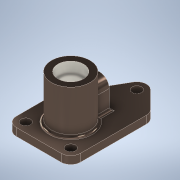
# Autodesk Inventor part: Part12. Pole Foot
Saved by Autodesk Inventor 2022.2 (Build 262287010, 287A)
## iProperties
Created: 2022-12-07
Part Number: Part12. Pole Foot
Material: Steel, Carbon
Document SubType Name: Modeling
Designer: User
Mass: 2300.87 g
Surface Area: 538.828 cm^2
Volume: 293.105 cm^3
Density: 7.85 g/cm^3
Appearance: Gunmetal - Antique Polished
Author: User
Autodesk Inventor part; units mm, degrees
ref_plane "YZ Plane" through (0, 0, 0) normal (1, 0, 0) x (0, 1, 0)
ref_plane "XZ Plane" through (0, 0, 0) normal (0, 1, 0) x (-1, 0, 0)
sketch "Sketch2" plane through (0, 0, 0) normal (0, 1, 0) x (-1, 0, 0)
  circle A0 centre (0, 0) radius 15
  line L0 (35, 50) -> (-35, 50)
  line L1 (-50, 35) -> (-50, -68)
  line L2 (50, -20.5218) -> (50, 35)
  circle A1 centre (-8, -95) radius 7.5
  arc A2 (-18.6066, -105.6066) -> (4.9904, -102.5) centre (-8, -95) ccw
  line L3 (-18.6066, -105.6066) -> (-45.6066, -78.6066)
  line L4 (-18.6066, -105.6066) -> (19.5772, -105.6066) construction
  line L5 (4.9904, -102.5) -> (47.9904, -28.0218)
  line L6 (4.9904, -102.5) -> (90.9904, -102.5) construction
  arc A3 (-50, -68) -> (-45.6066, -78.6066) centre (-35, -68) ccw
  arc A4 (47.9904, -28.0218) -> (50, -20.5218) centre (35, -20.5218) ccw
  arc A5 (-35, 50) -> (-50, 35) centre (-35, 35) ccw
  arc A6 (50, 35) -> (35, 50) centre (35, 35) ccw
  circle A7 centre (35, 35) radius 7.5
  circle A8 centre (-35, 35) radius 7.5
  dimension "d11" = 30
  dimension "d12" = 50
  dimension "d13" = 50
  dimension "d14" = 100
  dimension "d15" = 15
  dimension "d16" = 145
  dimension "d17" = 42
  dimension "d19" = 60
  dimension "d21" = 15
  dimension "d22" = 135
  dimension "d23" = 15
  dimension "d24" = 15
  dimension "d25" = 15
  constraints: 14 end point, 12 point on circle, 10 tangent, 9 centre point, 4 coincident, 3 equal radius, 3 horizontal, 2 equal length, 2 point on line, 1 parallel, 1 perpendicular
  measures "d11" diameter of A0
  measures "d12" distance from line of point (0, 0) L0
  measures "d13" distance from line of L2 point (0, 0)
  measures "d14" distance between parallel lines of L1 L2
  measures "d15" diameter of A1
  measures "d16" distance from line of A1.centre L0
  measures "d17" distance from line of L1 A1.centre
  measures "d19" angle of L6 L5
  measures "d21" radius of A2
  measures "d22" angle of L1 L3
  measures "d23" radius of A3
  measures "d24" diameter of A7
  measures "d25" diameter of A8
extrude "Extrusion1" add sketch "Sketch2" along normal blind 12
sketch "Sketch3" plane through (0, 12, 0) normal (0, 1, 0) x (1, 0, 0)
  circle A0 centre (0, 0) radius 15 projected
  line L0 (-4.9904, 102.5) -> (-47.9904, 28.0218) projected
  arc A1 (-47.9904, 28.0218) -> (-50, 20.5218) centre (-35, 20.5218) ccw projected
  line L1 (-50, 20.5218) -> (-50, -35) projected
  arc A2 (-50, -35) -> (-35, -50) centre (-35, -35) ccw projected
  line L2 (-35, -50) -> (35, -50) projected
  arc A3 (35, -50) -> (50, -35) centre (35, -35) ccw projected
  line L3 (50, -35) -> (50, 68) projected
  arc A4 (50, 68) -> (45.6066, 78.6066) centre (35, 68) ccw projected
  line L4 (45.6066, 78.6066) -> (18.6066, 105.6066) projected
  arc A5 (18.6066, 105.6066) -> (-4.9904, 102.5) centre (8, 95) ccw projected
  circle A6 centre (0, 0) radius 15 projected
  circle A7 centre (35, -35) radius 7.5 projected
  circle A8 centre (-35, -35) radius 7.5 projected
  circle A9 centre (8, 95) radius 7.5 projected
  circle A10 centre (0, 0) radius 30
  dimension "d28" = 60
  constraints: 1 centre point, 1 coincident
  measures "d28" diameter of A10
extrude "Extrusion2" add sketch "Sketch3" along normal blind 68 contours A10
sketch "Sketch4" plane through (0, 80, 0) normal (0, 1, 0) x (1, 0, 0)
  circle A0 centre (0, 0) radius 15 projected
  circle A1 centre (0, 0) radius 30 projected
  circle A2 centre (0, 0) radius 15 projected
  circle A3 centre (0, 0) radius 20
  dimension "d31" = 40
  constraints: 1 centre point, 1 coincident
  measures "d31" diameter of A3
extrude "Extrusion3" cut sketch "Sketch4" against normal blind 16 contours A3
ref_plane "Work Plane1" through (0, 0, -30) normal (0, 0, 1) x (1, 0, 0)
sketch "Sketch5" plane through (0, 0, -30) normal (0, 0, 1) x (1, 0, 0)
  line L0 (0, -16) -> (0, 96) construction
  line L1 (-70, 0) -> (70, 0) construction
  circle A0 centre (0, 42) radius 8
  arc A1 (15, 42) -> (-15, 42) centre (0, 42) ccw
  line L2 (-35, 0) -> (35, 0) projected
  line L3 (35, 0) -> (35, 12) projected
  line L4 (-35, 12) -> (35, 12) projected
  line L5 (-35, 0) -> (-35, 12) projected
  line L6 (15, 42) -> (15, 12)
  line L7 (-15, 42) -> (-15, 12)
  point P0 (0, 0)
  point P1 (0, 57)
  dimension "d35" = 16
  dimension "d36" = 42
  dimension "d37" = 15
  constraints: 4 end point, 4 point on line, 3 point on circle, 2 centre point, 2 perpendicular, 2 tangent, 1 coincident
  measures "d35" diameter of A0
  measures "d36" distance from line of L1 A0.centre
  measures "d37" radius of A1
extrude "Extrusion4" add sketch "Sketch5" along normal up to surface contours L6 L4 L7 A1 round surface about axis through (0, 12, 0) along (0, 1, 0) radius 30 far side no
sketch "Sketch6" plane through (0, 0, -30) normal (0, 0, -1) x (-1, 0, 0)
  arc A0 (0, 57) -> (-15, 42) centre (0, 42) ccw projected
  line L0 (-15, 12) -> (-15, 42) projected
  line L1 (15, 12) -> (-15, 12) projected
  line L2 (15, 42) -> (15, 12) projected
  arc A1 (15, 42) -> (0, 57) centre (0, 42) ccw projected
  arc A2 (0, 34) -> (0, 50) centre (0, 42) ccw projected
  arc A3 (0, 34) -> (0, 50) centre (0, 42) ccw projected
  point P0 (0, 0)
extrude "Extrusion5" add sketch "Sketch6" along normal blind 15
sketch "Sketch7" plane through (0, 0, -45) normal (0, 0, -1) x (-1, 0, 0)
  arc A0 (15, 42) -> (-15, 42) centre (0, 42) ccw projected
  arc A1 (15, 42) -> (-15, 42) centre (0, 42) ccw projected
  line L0 (-15, 42) -> (-15, 12) projected
  line L1 (15, 12) -> (-15, 12) projected
  line L2 (15, 12) -> (15, 42) projected
  point P0 (0, 0)
hole "Hole1" at (0, 42, -45) direction (0, 0, 1) diameter 16 end up to face face through (0, 0, 0) facing (0, 1, 0) round with radius 15 far side no
fillet "Fillet1" radius 4 5 edges at (25.9808, 12, -15) (-15, 12, 25.9808) (15, 12, -35.4904) (0, 12, -45) (-15, 12, -35.4904)
body "Solid1"
